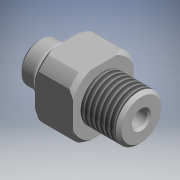
# Autodesk Inventor part: 007R000-0.725_rod_guide
Saved by Autodesk Inventor 2017.3 (Build 213256000, 256)
## iProperties
Part Number: 007R000-0.725_rod_guide
Material: Generic
Catalog Web Link: www.cadenas.de
Description: Rod Guide-Original Line - Standard Air Cylinders
Vendor: BIMBA
Document SubType Name: Modeling
Designer: partserver
Manufacturer: BIMBA
Mass: 1.83557 g
Surface Area: 13.2161 cm^2
Volume: 1.83557 cm^3
Density: 1 g/cm^3
Appearance: PSOLRGB-211-211-211
Category: PARTsolutions
Company: BIMBA
Title: 007R000-0.725_rod_guide
Author: Cadenas PARTsolutions
Comments: Original Line - Standard Air Cylinders
PSOL_IDENT_0: {$CADENAS_DATA\23d-libs\bimba\bimba_brand\bimba_imperial\bimba_full_line\original_line_cylinders\sta
PSOL_IDENT_1: ndard_air_cylinders\rod_guide.prj},261 {VTYP=3D},{NB=007R000-0.725_rod_guide},{LINA=007R000-0.725_ro
PSOL_IDENT_2: d_guide},{NN=Rod Guide},{DATE=19.01.2022 10:19:37},{GEOMDATE=12.08.2021 06:17:07},{VERSION=},{LINEID=
PSOL_IDENT_3: 10},{WBVAR=MNT,ACTING,NR,K,Q,T1,T2,T3,T4,MB,TRIM,CUSH,RODTRANS},{WBNUMERIC=MB,TRIM,CUSH,RODTRANS}  {
PSOL_IDENT_4: NB=007R000-0.725_rod_guide},{LINA=007R000-0.725_rod_guide},{KT=DUMMY},{PN=007R000},{BORE=0.31250000}
PSOL_IDENT_5: ,{BOREPN=007},{MNT=},{MNTALG='' , 'Front Nose' , 'BF' , 'Front Block'},{ACTING=R},{ACTINGALG= '' , '
PSOL_IDENT_6: Single Acting' , 'R' , 'Reverse/Double Acting' },{NR=},{NRALG= '' , 'N/A' },{K=},{Q=},{QALG= '' , 'W
PSOL_IDENT_7: ithout Side Ported Rear Head' , 'Q' , 'With Side Ported Rear Head' },{T1=},{T2=},{T3=},{T4=},{MB=0},
PSOL_IDENT_8: {A1=0.8450},{A1N=0.6250},{A1P=0.8450},{A1B=0.9060},{A2=0.3120},{A2N=0.2500},{A2P=0.3120},{A3=0.3125}
PSOL_IDENT_9: ,{A3N=0.1200},{A3P=0.3125},{A4=0.1585},{A4N=0.2550},{A4P=0.1585},{A5=0.0220},{A6=0.0000},{A6N=0.1025
PSOL_IDENT_10: },{A6P=0.0000},{A7=0.3040},{A7N=0.2050},{A7P=0.3040},{A8=0.0150},{A8N=0.0150},{A8NR=0.0150},{D1=0.60
PSOL_IDENT_11: 50},{D1N=0.3590},{D1P=0.6050},{D1B=0.0000},{D2=0.3215},{D3=0.0000},{D3N=0.2350},{D3P=0.0000},{D4=0.1
PSOL_IDENT_12: 530},{D4N=0.1420},{D4P=0.1530},{D4NR=0.1530},{D5=0.1280},{D5N=0.1280},{D5NR=0.1280},{C1=0.020},{C2=0
PSOL_IDENT_13: .0200},{C2N=0.0200},{C2P=0.0200},{C3=0.0300},{C3N=0.0000},{C3P=0.0300},{C4=0.0300},{C4N=0.0200},{C4P=
PSOL_IDENT_14: 0.0300},{NDM=0.3750},{NDMN=0.2500},{NDMP=0.3750},{TAB=UNF},{D6=0.0000},{D6N=0.0000},{D6P=0.0000},{A9=
PSOL_IDENT_15: 0.0000},{A9N=0.0000},{A9P=0.0000},{D7=0.0000},{D7N=0.0000},{D7P=0.0000},{A10=0.0000},{A10N=0.0000},{
PSOL_IDENT_16: A10P=0.0000},{R1=0.0000},{R1N=0.0000},{R1P=0.0000},{D8=0.0000},{D9=0.0000},{D10=0.0000},{A11=0.0000}
PSOL_IDENT_17: ,{A12=0.0000},{A13=0.0000},{A14=0.3750},{A14N=0.3750},{A14B=0.5000},{D11=0.0000},{D11N=0.0000},{NDM2=
PSOL_IDENT_18: 0.1900},{NDM2N=0.1900},{NDM2DP=0.0000},{THREAD=1},{HEX=0.0000},{HEXN=0.0000},{S1=0.5000},{B1=0.0620}
PSOL_IDENT_19: ,{B2=0.5940},{B22=0.0000},{DB=0.1130},{B3=0.0150},{B4=0.3430},{X1=0.0000},{X2=0.0000},{NDM3=0.0000},
PSOL_IDENT_20: {NDM4=0.0000},{NDM4DP=0.0000},{DD=0.0000},{CB=0.0000},{CBDP=0.0000},{PORT=1},{XT=0.0000},{XTX=0.0000
PSOL_IDENT_21: },{XT1=0.0000},{XT2=0.0000},{NDMH=0.0000},{OD=0.3590},{ID=0.3215},{G=0.0000},{PNUT=0.3120},{TRIM=0},
PSOL_IDENT_22: {C11=0.0000},{C22=0.0000},{C33=0.0000},{C44=0.0000},{C55=0.0000},{CD1=0.0000},{CD2=0.0000},{CD3=0.00
PSOL_IDENT_23: 00},{CNDM3=0.0000},{CTAB3=0.0000},{CUSH=0},{XX=0.34300},{LCD=0.0000},{RODTRANS=0.72500}
NB: 007R000-0.725_rod_guide
NN: Rod Guide
NT: Original Line - Standard Air Cylinders
NBSYN: $PN.-$RODTRANS._rod_guide
LINA: 007R000-0.725_rod_guide
CATALOG: Bimba Products
BORE: 0
BOREPN: 007
MNT: Front Nose
MNTALG: '' , 'Front Nose' , 'BF' , 'Front Block'
ACTING: Reverse/Double Acting
NR: N/A
K: Standard
Q: Without Side Ported Rear Head
T1: without T1
T2: without T2
T3: without T3
T4: without T4
MB: 0
A1N: 0.625
A1P: 0.845
A1B: 0.906
A2N: 0.25
A2P: 0.312
A3N: 0.12
A3P: 0.3125
A4N: 0.255
A4P: 0.1585
A5: 0.022
A6N: 0.1025
A6P: 0
A7N: 0.205
A7P: 0.304
A8N: 0.015
A8NR: 0.015
D1N: 0.359
D1P: 0.605
D1B: 0
D2: 0.3215
D3N: 0.235
D3P: 0
D4N: 0.142
D4P: 0.153
D4NR: 0.153
D5N: 0.128
D5NR: 0.128
C1: 0.02
C2N: 0.02
C2P: 0.02
C3N: 0
C3P: 0.03
C4N: 0.02
C4P: 0.03
NDMN: 0.25
NDMP: 0.375
TAB: UNF
D6N: 0
D6P: 0
A9N: 0
A9P: 0
D7N: 0
D7P: 0
A10N: 0
A10P: 0
R1N: 0
R1P: 0
D8: 0
D9: 0
D10: 0
A11: 0
A12: 0
A13: 0
A14N: 0.375
A14B: 0.5
D11N: 0
NDM2N: 0.19
NDM2DP: 0
HEXN: 0
S1: 0.5
B1: 0.062
B2: 0.594
B22: 0
DB: 0.113
B3: 0.015
B4: 0.343
X1: 0
X2: 0
NDM3: 0
NDM4: 0
NDM4DP: 0
DD: 0
CB: 0
CBDP: 0
XTX: 0
XT1: 0
XT2: 0
NDMH: 0
TRIM: 0
C11: 0
C22: 0
C33: 0
C44: 0
C55: 0
CD1: 0
CD2: 0
CD3: 0
CNDM3: 0
CTAB3: 0.0000
CUSH: 0
LCD: 0
RODTRANS: 0.725
SUPPLIER: BIMBA
ARTICLENO: 007R000-0.725_rod_guide
BOMINFO: 007R000-0.725_rod_guide
CREATOR: CADENAS GmbH
Autodesk Inventor part; units mm, degrees
sketch "Sketch_1" plane through (0, 0, 0) normal (0, 0, 1) x (1, 0, 0)
  line L0 (7.9248, 0) -> (0, 0)
  line L1 (0, 0) -> (0, 4.1326)
  line L2 (0, 4.1326) -> (0.6299, 4.7625)
  line L3 (0.6299, 4.7625) -> (7.9248, 4.7625)
  line L4 (7.9248, 4.7625) -> (7.9248, 0)
  line L5 (7.9248, 0) -> (0, 0)
  constraints: 12 end point
revolve "Revolution1" add sketch "Sketch_1" angle 360 about axis through (7.9248, 0, 0) along (1, 0, 0)
thread "Thread1" size "3/8-24 UNF" class "2A" standard "ANSI Unified Screw Threads" full length
sketch "Sketch_3" plane through (0, 0, 0) normal (0, 0, 1) x (1, 0, 0)
  line L0 (21.463, 0) -> (7.9248, 0)
  line L1 (7.9248, 0) -> (7.9248, 6.9215)
  line L2 (7.9248, 6.9215) -> (8.6868, 7.6835)
  line L3 (8.6868, 7.6835) -> (15.1003, 7.6835)
  line L4 (15.1003, 7.6835) -> (15.8623, 6.9215)
  line L5 (15.8623, 6.9215) -> (15.8623, 3.5243)
  line L6 (15.8623, 3.5243) -> (17.9959, 3.5243)
  line L7 (17.9959, 3.5243) -> (18.5547, 4.0831)
  line L8 (18.5547, 4.0831) -> (20.955, 4.0831)
  line L9 (20.955, 4.0831) -> (21.463, 3.575)
  line L10 (21.463, 3.575) -> (21.463, 0)
  line L11 (21.463, 0) -> (7.9248, 0)
  constraints: 24 end point
revolve "Revolution2" add sketch "Sketch_3" angle 360 about axis through (21.463, 0, 0) along (1, 0, 0)
sketch "Sketch_17" plane through (0, 0, 0) normal (0, 0, 1) x (1, 0, 0)
  line L0 (17.4371, 0) -> (15.8623, 0)
  line L1 (15.8623, 0) -> (15.8623, 4.5593)
  line L2 (15.8623, 4.5593) -> (17.4371, 4.5593)
  line L3 (17.4371, 4.5593) -> (17.4371, 0)
  line L4 (17.4371, 0) -> (15.8623, 0)
  constraints: 10 end point
revolve "Revolution3" add sketch "Sketch_17" angle 360 about axis through (17.4371, 0, 0) along (1, 0, 0)
sketch "Sketch4" plane through (0, 0, 0) normal (-1, 0, 0) x (0, 0, 1)
  point P0 (0, 0)
hole "Hole1" at (0, 0, 0) direction (1, 0, 0) diameter 3.2512 depth 21.463 countersink diameter 4.0132 countersink angle 90
sketch "Sketch_16" plane through (0, 0, 0) normal (1, 0, 0) x (0, 1, 0)
  line L0 (-12.7, 12.7) -> (-12.7, -12.7)
  line L1 (-12.7, -12.7) -> (12.7, -12.7)
  line L2 (12.7, -12.7) -> (12.7, 12.7)
  line L3 (12.7, 12.7) -> (-12.7, 12.7)
  line L4 (-6.35, 6.35) -> (-6.35, -6.35)
  line L5 (-6.35, -6.35) -> (6.35, -6.35)
  line L6 (6.35, -6.35) -> (6.35, 6.35)
  line L7 (6.35, 6.35) -> (-6.35, 6.35)
  constraints: 16 end point
extrude "Extrusion1" cut sketch "Sketch_16" along normal blind 21.463
sketch "Sketch6" plane through (8.6868, -4.3259, 6.35) normal (0, 0, 1) x (1, 0, 0)
  point P0 (3.2512, 4.3259)
hole "Hole2" at (11.938, 0, 6.35) direction (0, 0, -1) diameter 3.9624 depth 6.35 countersink diameter 4.826 countersink angle 90 thread size "10-32 UNF" class "2B" standard "ANSI Unified Screw Threads"
sketch "Sketch_47" plane through (0, 0, 0) normal (0, 0, 1) x (1, 0, 0)
  line L0 (17.9959, 0) -> (17.4371, 0)
  line L1 (17.4371, 4.0431) -> (17.4371, 3.2702)
  line L2 (17.4371, 3.2702) -> (17.9959, 3.2702)
  line L3 (17.9959, 3.2702) -> (17.9959, 3.5243)
  line L4 (17.9959, 3.5243) -> (17.7165, 3.5243)
  line L5 (17.7165, 3.5243) -> (17.5509, 3.6899)
  arc A0 (17.5509, 3.8695) -> (17.5509, 3.6899) centre (17.6407, 3.7797) ccw
  line L6 (17.5509, 3.8695) -> (18.1565, 4.4751)
  line L7 (18.1565, 4.4751) -> (18.1565, 4.5593)
  line L8 (18.1565, 4.5593) -> (17.9533, 4.5593)
  line L9 (17.9533, 4.5593) -> (17.4371, 4.0431)
  constraints: 20 end point, 2 point on circle, 1 centre point
revolve "Revolution4" add sketch "Sketch_47" angle 360 about axis through (17.9959, 0, 0) along (1, 0, 0)
ref_plane "hh_XY" through (0, 4.7625, 0) normal (0, 0, 1) x (1, 0, 0)
ref_plane "hh_YZ" through (0, 4.7625, 0) normal (1, 0, 0) x (0, 1, 0)
ref_plane "hh_ZX" through (0, 4.7625, 0) normal (0, 1, 0) x (0, 0, 1)
ref_plane "port_XY" through (11.938, 0, 0) normal (0, 0, 1) x (1, 0, 0)
ref_plane "port_YZ" through (11.938, 0, 0) normal (1, 0, 0) x (0, 1, 0)
ref_plane "port_ZX" through (11.938, 0, 0) normal (0, 1, 0) x (0, 0, 1)
ref_plane "rod_guide_XY" through (0, 0, 0) normal (1, 0, 0) x (0, 0, -1)
ref_plane "rod_guide_YZ" through (0, 0, 0) normal (0, 0, -1) x (0, 1, 0)
ref_plane "rod_guide_ZX" through (0, 0, 0) normal (0, 1, 0) x (1, 0, 0)
ref_plane "sq1_XY" through (0, 0, 6.35) normal (1, 0, 0) x (0, 0, -1)
ref_plane "sq1_YZ" through (0, 0, 6.35) normal (0, 0, -1) x (0, 1, 0)
ref_plane "sq1_ZX" through (0, 0, 6.35) normal (0, 1, 0) x (1, 0, 0)
ref_plane "sq2_XY" through (0, 0, -6.35) normal (1, 0, 0) x (0, 0, -1)
ref_plane "sq2_YZ" through (0, 0, -6.35) normal (0, 0, -1) x (0, 1, 0)
ref_plane "sq2_ZX" through (0, 0, -6.35) normal (0, 1, 0) x (1, 0, 0)
ref_plane "t1_XY" through (7.9248, 0, 0) normal (1, 0, 0) x (0, 0, -1)
ref_plane "t1_YZ" through (7.9248, 0, 0) normal (0, 0, -1) x (0, 1, 0)
ref_plane "t1_ZX" through (7.9248, 0, 0) normal (0, 1, 0) x (1, 0, 0)
ref_plane "t111_XY" through (7.9248, 0, 0) normal (1, 0, 0) x (0, 0, -1)
ref_plane "t111_YZ" through (7.9248, 0, 0) normal (0, 0, -1) x (0, 1, 0)
ref_plane "t111_ZX" through (7.9248, 0, 0) normal (0, 1, 0) x (1, 0, 0)
ref_plane "to_foot_bracket_XY" through (7.9248, 0, 0) normal (1, 0, 0) x (0, 0, -1)
ref_plane "to_foot_bracket_YZ" through (7.9248, 0, 0) normal (0, 0, -1) x (0, 1, 0)
ref_plane "to_foot_bracket_ZX" through (7.9248, 0, 0) normal (0, 1, 0) x (1, 0, 0)
ref_plane "to_nut_XY" through (7.9248, 0, 0) normal (1, 0, 0) x (0, 0, -1)
ref_plane "to_nut_YZ" through (7.9248, 0, 0) normal (0, 0, -1) x (0, 1, 0)
ref_plane "to_nut_ZX" through (7.9248, 0, 0) normal (0, 1, 0) x (1, 0, 0)
ref_plane "to_rod_XY" through (-18.415, 0, 0) normal (1, 0, 0) x (0, 0, -1)
ref_plane "to_rod_YZ" through (-18.415, 0, 0) normal (0, 0, -1) x (0, 1, 0)
ref_plane "to_rod_ZX" through (-18.415, 0, 0) normal (0, 1, 0) x (1, 0, 0)
ref_plane "to_screw_XY" through (11.938, 0, 0) normal (0, 1, 0) x (1, 0, 0)
ref_plane "to_screw_YZ" through (11.938, 0, 0) normal (1, 0, 0) x (0, 0, -1)
ref_plane "to_screw_ZX" through (11.938, 0, 0) normal (0, 0, -1) x (0, 1, 0)
ref_plane "to_trunnion_brackets_XY" through (0, 0, 0) normal (0, 1, 0) x (1, 0, 0)
ref_plane "to_trunnion_brackets_YZ" through (0, 0, 0) normal (1, 0, 0) x (0, 0, -1)
ref_plane "to_trunnion_brackets_ZX" through (0, 0, 0) normal (0, 0, -1) x (0, 1, 0)
ref_plane "to_trunnion_brackets1_XY" through (0, 6.35, 0) normal (0, 1, 0) x (1, 0, 0)
ref_plane "to_trunnion_brackets1_YZ" through (0, 6.35, 0) normal (1, 0, 0) x (0, 0, -1)
ref_plane "to_trunnion_brackets1_ZX" through (0, 6.35, 0) normal (0, 0, -1) x (0, 1, 0)
ref_plane "to_trunnion_brackets2_XY" through (0, -6.35, 0) normal (0, 1, 0) x (1, 0, 0)
ref_plane "to_trunnion_brackets2_YZ" through (0, -6.35, 0) normal (1, 0, 0) x (0, 0, -1)
ref_plane "to_trunnion_brackets2_ZX" through (0, -6.35, 0) normal (0, 0, -1) x (0, 1, 0)
ref_plane "to_tube_XY" through (17.9959, 0, 0) normal (1, 0, 0) x (0, 0, -1)
ref_plane "to_tube_YZ" through (17.9959, 0, 0) normal (0, 0, -1) x (0, 1, 0)
ref_plane "to_tube_ZX" through (17.9959, 0, 0) normal (0, 1, 0) x (1, 0, 0)
body "Solid1"
